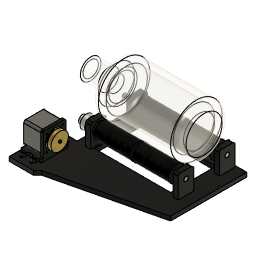
ball-mill v9 (Autodesk Fusion 360 design; units mm, degrees)
Autodesk Fusion 360 part; units mm, degrees
sketch "Sketch1" plane through (0, 0, 0) normal (1, 0, 0) x (0, 1, 0)
  line L0 (17, -21) -> (-17, -21)
  line L1 (-21, -17) -> (-21, 17)
  line L2 (-17, 21) -> (17, 21)
  line L3 (21, 17) -> (21, -17)
  line L4 (21, -21) -> (-21, 21) construction
  line L5 (-21, -21) -> (21, 21) construction
  line L6 (15.5, -15.5) -> (-15.5, -15.5)
  line L7 (-15.5, -15.5) -> (-15.5, 15.5)
  line L8 (-15.5, 15.5) -> (15.5, 15.5)
  line L9 (15.5, 15.5) -> (15.5, -15.5)
  line L10 (15.5, -15.5) -> (-15.5, 15.5) construction
  line L11 (-15.5, -15.5) -> (15.5, 15.5) construction
  circle A0 centre (-15.5, 15.5) radius 1.5
  circle A1 centre (-15.5, -15.5) radius 1.5
  circle A2 centre (15.5, -15.5) radius 1.5
  circle A3 centre (15.5, 15.5) radius 1.5
  arc A4 (-17, 21) -> (-21, 17) centre (-17, 17) ccw
  arc A5 (21, 17) -> (17, 21) centre (17, 17) ccw
  arc A6 (17, -21) -> (21, -17) centre (17, -17) ccw
  arc A7 (-21, -17) -> (-17, -21) centre (-17, -17) ccw
  circle A8 centre (0, 0) radius 11
  circle A9 centre (0, 0) radius 2.5
  dimension "d1" = 42
  dimension "d2" = 42
  dimension "d3" = 31
  dimension "d4" = 3
  dimension "d6" = 360
  dimension "d7" = 4
  dimension "d8" = 22
  dimension "d9" = 5
  constraint horizontal L0
  constraint perpendicular L0 L1
  constraint parallel L0 L2
  constraint parallel L1 L3
  constraint coincident L4 A8.centre
  constraint coincident L5 A8.centre
  constraint coincident A8.centre A9.centre
  constraint horizontal L6
  constraint perpendicular L6 L7
  constraint parallel L6 L8
  constraint parallel L7 L9
  constraint coincident L10 A8.centre
  constraint coincident L11 A8.centre
  constraint coincident L4 L6.start
  constraint coincident L7.end L8.start
  constraint coincident L4.end L2
  constraint coincident L4.end L1
  constraint tangent L2 A4
  constraint tangent L1 A4
  constraint coincident L5.end L2
  constraint coincident L5.end L3
  constraint tangent L2 A5
  constraint tangent L3 A5
  constraint equal A4 A5
  constraint coincident L4.start L3
  constraint coincident L4.start L0
  constraint tangent L3 A6
  constraint tangent L0 A6
  constraint equal A4 A6
  constraint coincident L5.start L0
  constraint coincident L5.start L1
  constraint tangent L0 A7
  constraint tangent L1 A7
  constraint equal A4 A7
  constraint concentric A8 A9
  measures "d1" distance of L4.end L5.end
  measures "d2" distance of L4.start L5.end
  measures "d3" distance of L7.end L8.end
  measures "d4" diameter of A0
  measures "d7" radius of A4
  measures "d8" diameter of A8
  measures "d9" diameter of A9
  measures "d130" radius of L8.end
extrude "Extrude1" add sketch "Sketch1" against normal blind 34 contours L0 L1 L2 L3 A4 A5 A6 A7 | L6 L7 A1 | L6 L7 L8 L9 A0 A1 A2 A3 | L6 L7 A1 | L6 L9 A2 | L6 L9 A2 | L7 L8 A0 | L7 L8 A0 | L8 L9 A3 | L8 L9 A3 | A8 | A9 makes body 1
extrude "Extrude2" cut sketch "Sketch1" against normal blind 5 contours L6 L7 A1 | L6 L7 A1 | L6 L9 A2 | L6 L9 A2 | L7 L8 A0 | L7 L8 A0 | L8 L9 A3 | L8 L9 A3 bodies 1
extrude "Extrude3" add sketch "Sketch1" along normal blind 2 contours A8 | A9 bodies 1
extrude "Extrude4" add sketch "Sketch1" along normal blind 17 contours A9 bodies 1
chamfer "Chamfer1" distance 0.5 angle 45 1 edges at (17, -2.3308, -0.904) on bodies 1
sketch "Sketch2" plane through (0, 0, 0) normal (1, 0, 0) x (0, 1, 0)
  line L0 (22, -22.25) -> (-22, -22.25)
  line L1 (-22, -22.25) -> (-22, 20.25)
  line L2 (-20, 22.25) -> (20, 22.25)
  line L3 (22, 20.25) -> (22, -22.25)
  line L4 (22, -22.25) -> (-22, 22.25) construction
  line L5 (-22, -22.25) -> (22, 22.25) construction
  line L6 (0, 0) -> (-15.5, 15.5) construction
  line L7 (-15.5, -15.5) -> (15.5, 15.5) construction
  circle A0 centre (-15.5, 15.5) radius 1.7
  circle A1 centre (-15.5, -15.5) radius 1.7
  circle A2 centre (15.5, -15.5) radius 1.7
  circle A3 centre (15.5, 15.5) radius 1.7
  circle A4 centre (0, 0) radius 17.5
  line L8 (20, 22.25) -> (22, 20.25)
  line L9 (-22, 20.25) -> (-20, 22.25)
  line L10 (0, -28.25) -> (34, -28.25)
  line L11 (34, -28.25) -> (34, -22.25)
  line L12 (34, -22.25) -> (22, -22.25)
  line L13 (0, -28.25) -> (-34, -28.25)
  line L14 (-34, -22.25) -> (-22, -22.25)
  line L15 (-34, -28.25) -> (-34, -22.25)
  dimension "d19" = 44
  dimension "d20" = 44.5
  dimension "d21" = 31
  dimension "d22" = 3.4
  dimension "d24" = 360
  dimension "d25" = 35
  dimension "d26" = 2
  dimension "d27" = 2
  dimension "d28" = 2
  dimension "d29" = 2
  dimension "d35" = 6
  dimension "d36" = 34
  dimension "d37" = 12
  constraint horizontal L0
  constraint perpendicular L0 L1
  constraint parallel L0 L2
  constraint parallel L1 L3
  constraint coincident L4 L6.start
  constraint coincident L5 L6.start
  constraint coincident L6.start A4.centre
  constraint coincident L6 A4.centre
  constraint coincident L7 L6.start
  constraint coincident L6.end A0.centre
  constraint coincident L5.end L2
  constraint coincident L5.end L3
  constraint coincident L4.end L1
  constraint coincident L4.end L2
  constraint parallel L0 L10
  constraint perpendicular L10 L11
  constraint perpendicular L3 L12
  measures "d19" distance of L4.end L5.end
  measures "d20" distance of L0.end L4.end
  measures "d21" distance of L6.end L7.end
  measures "d22" diameter of A0
  measures "d25" diameter of A4
  measures "d26" distance of L5.end L2.end
  measures "d27" distance of L5.end L3.start
  measures "d28" distance of L4.end L1.end
  measures "d29" distance of L4.end L2.start
  measures "d35" distance of L10.end L11.end
  measures "d36" distance of L10.start L10.end
  measures "d37" distance of L0.start L11.end
ref_plane "WorkPlane1" through (15, 0, 0) normal (1, 0, 0) x (0, 1, 0)
sketch "Sketch3" plane through (15, 0, 0) normal (1, 0, 0) x (0, 1, 0)
  circle A0 centre (0, 0) radius 16.9
  circle A1 centre (0, 0) radius 2.5
  dimension "d31" = 33.8
  dimension "d34" = 5
  constraint coincident A0.centre A1.centre
  measures "d31" diameter of A0
  measures "d34" diameter of A1
extrude "Extrude5" add sketch "Sketch3" against normal blind 7 separate body makes body 2
extrude "Extrude6" add sketch "Sketch2" along normal blind 5 separate body contours L0 L1 L2 L3 L8 L9 makes body 3
extrude "Extrude7" add sketch "Sketch2" along normal blind 5 and the other way blind 34 contours L0 L10 L11 L12 L13 L14 L15 bodies 3
sketch "Sketch4" plane through (0, 0, -22.25) normal (0, 0, 1) x (-1, 0, 0)
  line L0 (0, -22) -> (-5, -22)
  line L1 (-5, -22) -> (-5, -34)
  line L2 (-5, -34) -> (34, -34)
  line L3 (34, -34) -> (34, 34)
  line L4 (34, 34) -> (-5, 34)
  line L5 (-5, 34) -> (-5, 22)
  line L6 (-5, 22) -> (0, 22)
  line L7 (0, 22) -> (0, -22)
  line L8 (-5, -22) -> (34, -22)
  line L9 (34, -22) -> (34, -34)
  line L10 (34, -34) -> (-5, -34)
  line L11 (-5, -34) -> (-5, -26)
  line L12 (5, 0) -> (6, 0)
  line L13 (6, 0) -> (19, 0)
  line L14 (9, -30) -> (9, -29)
  line L15 (12, -26) -> (18, -26)
  line L16 (21, -30) -> (21, -29)
  line L17 (1, -30) -> (1, -29)
  line L18 (-2, -26) -> (-5, -26)
  line L19 (29, -30) -> (29, -29)
  line L20 (32, -26) -> (34, -26)
  circle A0 centre (5, -30) radius 2.25
  circle A1 centre (25, -30) radius 2.25
  arc A2 (1, -30) -> (9, -30) centre (5, -30) ccw
  arc A3 (21, -30) -> (29, -30) centre (25, -30) ccw
  line L21 (25, -34) -> (25, -39)
  line L22 (-5, -34) -> (34, -34)
  line L23 (34, -26) -> (34, -34)
  arc A4 (1, -29) -> (-2, -26) centre (-2, -29) ccw
  arc A5 (12, -26) -> (9, -29) centre (12, -29) ccw
  arc A6 (21, -29) -> (18, -26) centre (18, -29) ccw
  arc A7 (32, -26) -> (29, -29) centre (32, -29) ccw
  line L24 (-5, 34) -> (34, 34)
  line L25 (0, 22) -> (-5, 22)
  line L26 (-5, 22) -> (-5, 34)
  line L27 (-5, 22) -> (34, 22)
  arc A8 (9, 30) -> (1, 30) centre (5, 30) ccw
  line L28 (21, 30) -> (21, 29)
  line L29 (34, 26) -> (34, 34)
  line L30 (1, 30) -> (1, 29)
  arc A9 (18, 26) -> (21, 29) centre (18, 29) ccw
  line L31 (29, 30) -> (29, 29)
  arc A10 (29, 29) -> (32, 26) centre (32, 29) ccw
  line L32 (9, 30) -> (9, 29)
  line L33 (12, 26) -> (18, 26)
  line L34 (34, 22) -> (34, 34)
  arc A11 (9, 29) -> (12, 26) centre (12, 29) ccw
  line L35 (-2, 26) -> (-5, 26)
  line L36 (34, 34) -> (-5, 34)
  line L37 (-5, 34) -> (-5, 26)
  line L38 (-5, 34) -> (34, 34)
  circle A12 centre (5, 30) radius 2.25
  circle A13 centre (25, 30) radius 2.25
  arc A14 (-2, 26) -> (1, 29) centre (-2, 29) ccw
  line L39 (32, 26) -> (34, 26)
  arc A15 (29, 30) -> (21, 30) centre (25, 30) ccw
  point P0 (25, 34)
  dimension "d47" = 4.5
  dimension "d48" = 4.5
  dimension "d49" = 3
  constraint horizontal L8
  constraint vertical L9
  constraint horizontal L10
  constraint vertical L11
  constraint coincident L2.end L3.start
  constraint coincident L0.end L1.start
  constraint perpendicular L7 L12
  constraint perpendicular L7 L13
  constraint tangent L10 A2
  constraint tangent L2 A3
  constraint tangent L14 A2
  constraint tangent L16 A3
  constraint tangent L17 A2
  constraint perpendicular L11 L18
  constraint tangent L19 A3
  constraint coincident L9 L20.end
  constraint concentric A0 A2
  constraint concentric A1 A3
  constraint coincident L2 L21.start
  constraint tangent L18 A4
  constraint tangent L17 A4
  constraint tangent L15 A5
  constraint tangent L14 A5
  constraint equal A4 A5
  constraint tangent L15 A6
  constraint tangent L16 A6
  constraint equal A4 A6
  constraint tangent L19 A7
  constraint tangent L20 A7
  constraint equal A4 A7
  constraint symmetric L0.start L13 L6.end
  constraint symmetric L0.end L13 L5.end
  constraint symmetric L1.end L13 L4.end
  constraint symmetric L2.end L13 L3.end
  constraint symmetric L8.end L13 L27.end
  constraint symmetric L13 L14.start A8.start
  constraint symmetric L13 L16.start L28.start
  constraint symmetric L13 L17.start A8.end
  constraint symmetric L13 L11.end L35.end
  constraint symmetric L13 L19.start L31.start
  constraint symmetric L13 L20.end L29.start
  constraint symmetric L13 A0 A12
  constraint symmetric L13 A1 A13
  constraint symmetric L13 A2 A8
  constraint symmetric L13 A3 A15
  constraint symmetric L13 L21.start P0
  constraint symmetric L13 L18.start L35.start
  constraint symmetric L13 L17.end L30.end
  constraint symmetric L13 A4 A14
  constraint symmetric L13 L15.start L33.start
  constraint symmetric L13 L14.end L32.end
  constraint symmetric L13 A5 A11
  constraint symmetric L13 L15.end A9.start
  constraint symmetric L13 L16.end L28.end
  constraint symmetric L13 A6 A9
  constraint symmetric L13 L19.end L31.end
  constraint symmetric L13 L20.start A10.end
  constraint symmetric L13 A7 A10
  measures "d47" diameter of A0
  measures "d48" diameter of A1
  measures "d49" radius of A4
extrude "Extrude8" cut sketch "Sketch4" against normal blind 10 contours L1 L2 L10 L11 L17 L18 A2 L22 A4 | L2 L3 L9 L10 L19 L20 A3 L22 L23 A7 | L4 L5 L24 L26 A8 L30 L35 L36 L37 L38 A14 | L3 L4 L24 L29 L31 A10 L34 L36 L38 L39 A15 | L2 L10 L14 L15 L16 A2 A3 L22 A5 A6 | L4 L24 A8 L28 A9 L32 L33 A11 L36 L38 A15 bodies 3
extrude "Extrude9" cut sketch "Sketch4" against normal blind 10 contours A0 | A1 | A12 | A13 bodies 3
sketch "Sketch5" plane through (0, 0, -28.25) normal (0, 0, -1) x (1, 0, 0)
  circle A0 centre (-25, -30) radius 2.25
  circle A1 centre (-25, 30) radius 2.25
  circle A2 centre (-5, -30) radius 2.25
  circle A3 centre (-5, 30) radius 2.25
  line L0 (5, 26) -> (2, 26)
  arc A4 (-1, 29) -> (2, 26) centre (2, 29) ccw
  line L1 (-1, 29) -> (-1, 30)
  arc A5 (-1, 30) -> (-9, 30) centre (-5, 30) ccw
  line L2 (-9, 30) -> (-9, 29)
  arc A6 (-12, 26) -> (-9, 29) centre (-12, 29) ccw
  line L3 (-12, 26) -> (-18, 26)
  arc A7 (-21, 29) -> (-18, 26) centre (-18, 29) ccw
  line L4 (-21, 29) -> (-21, 30)
  arc A8 (-21, 30) -> (-29, 30) centre (-25, 30) ccw
  line L5 (-29, 30) -> (-29, 29)
  arc A9 (-32, 26) -> (-29, 29) centre (-32, 29) ccw
  line L6 (-32, 26) -> (-34, 26)
  line L7 (-34, 26) -> (-34, -26)
  line L8 (-34, -26) -> (-32, -26)
  arc A10 (-29, -29) -> (-32, -26) centre (-32, -29) ccw
  line L9 (-29, -29) -> (-29, -30)
  arc A11 (-29, -30) -> (-21, -30) centre (-25, -30) ccw
  line L10 (-21, -30) -> (-21, -29)
  arc A12 (-18, -26) -> (-21, -29) centre (-18, -29) ccw
  line L11 (-18, -26) -> (-12, -26)
  arc A13 (-9, -29) -> (-12, -26) centre (-12, -29) ccw
  line L12 (-9, -29) -> (-9, -30)
  arc A14 (-9, -30) -> (-1, -30) centre (-5, -30) ccw
  line L13 (-1, -30) -> (-1, -29)
  arc A15 (2, -26) -> (-1, -29) centre (2, -29) ccw
  line L14 (2, -26) -> (5, -26)
  line L15 (5, -26) -> (5, 26)
  line L16 (10, 38.1111) -> (-37, 38.1111)
  line L17 (-37, 38.1111) -> (-37, -37.8889)
  line L18 (-37, -37.8889) -> (10, -37.8889)
  line L19 (10, -37.8889) -> (10, 38.1111)
  line L20 (10, 38.1111) -> (-37, -37.8889) construction
  line L21 (-37, 38.1111) -> (10, -37.8889) construction
  line L22 (10, 38.1111) -> (17.9924, 38.1111)
  line L23 (220, -10) -> (220, -157.8889)
  line L24 (220, -157.8889) -> (10, -157.8889)
  line L25 (2.9501, -37.8889) -> (2.9501, -157.8889)
  line L26 (10, -157.8889) -> (2.9501, -157.8889)
  line L27 (-37, -37.8889) -> (-37, -45.8889)
  line L28 (-37, -45.8889) -> (2.9501, -45.8889)
  line L29 (-37, 38.1111) -> (-37, 46.1111)
  line L30 (-37, 46.1111) -> (10, 46.1111)
  line L31 (10, 46.1111) -> (17.9924, 38.1111)
  line L32 (220, -10) -> (17.9924, 38.1111)
  line L33 (180, -137.8889) -> (32.9501, -137.8889)
  line L34 (32.9501, -137.8889) -> (32.9501, -50)
  line L35 (32.9501, -50) -> (180, -50)
  line L36 (180, -50) -> (180, -137.8889)
  point P0 (-13.5, 0.1111)
  point P1 (-5, -30)
  dimension "d54" = 76
  dimension "d55" = 47
  dimension "d61" = 120
  dimension "d110" = 8
  dimension "d112" = 8
  dimension "d123" = 20
  dimension "d124" = 40
  dimension "d125" = 30
  dimension "d126" = 40
  dimension "d134" = 210
  constraint horizontal L16
  constraint perpendicular L16 L17
  constraint parallel L16 L18
  constraint parallel L17 L19
  constraint coincident L20 P0
  constraint coincident L21 P0
  constraint perpendicular L19 L22
  constraint perpendicular L22 L23
  constraint perpendicular L23 L24
  constraint coincident L18 L25.start
  constraint perpendicular L18 L25
  constraint perpendicular L18 L27
  constraint coincident L25 L28.end
  constraint perpendicular L25 L28
  constraint perpendicular L16 L29
  constraint perpendicular L29 L30
  constraint horizontal L33
  constraint vertical L34
  constraint horizontal L35
  constraint vertical L36
  measures "d54" distance of L16.end L17.end
  measures "d55" distance of L17.end L18.end
  measures "d61" distance of L18.end L24.end
  measures "d110" distance of L17.end L27.end
  measures "d112" distance of L16.end L29.end
  measures "d123" distance of L24 L33
  measures "d124" distance of L23.start L35
  measures "d125" distance of L25 L34
  measures "d126" distance of L23 L36
  measures "d134" distance of L23.end L24.end
extrude "Extrude10" add sketch "Sketch5" along normal blind 8 separate body contours L0 A4 L1 A5 L2 A6 L3 A7 L4 A8 L5 A9 L6 L7 L8 A10 L9 A11 L10 A12 L11 A13 L12 A14 L13 A15 L14 L15 | L16 L17 L18 L19 | L18 L19 L22 L23 L24 L25 L26 L32 | L16 L22 L29 L30 L31 | L18 L25 L27 L28 makes body 4
sketch "Sketch6" plane through (0, 0, -28.25) normal (0, 0, 1) x (-1, 0, 0)
  circle A0 centre (25, 30) radius 2.25
  circle A1 centre (5, 30) radius 2.25
  circle A2 centre (5, -30) radius 2.25
  circle A3 centre (25, -30) radius 2.25
  line L0 (-220, -10) -> (-220, -157.8889)
  line L1 (-220, -157.8889) -> (-2.9501, -157.8889)
  line L2 (-2.9501, -157.8889) -> (-2.9501, -45.8889)
  line L3 (37, -45.8889) -> (37, 46.1111)
  line L4 (-35, 0) -> (10, 0)
  line L5 (-230, -60) -> (70, -60)
  line L6 (-235, -110) -> (40, -110)
  line L7 (-15, 0) -> (-15, -175)
  line L8 (-8, -37.8889) -> (-8, -175)
  line L9 (-15, -60) -> (-35, -60)
  line L10 (-30, -60) -> (-30, -45)
  line L11 (-30, -45) -> (-20, -45)
  line L12 (-20, -45) -> (-20, -60)
  line L13 (-30, -60) -> (-30, -75)
  line L14 (-30, -75) -> (-20, -75)
  line L15 (-20, -75) -> (-20, -60)
  line L16 (-235.1894, -85) -> (34.547, -85)
  line L17 (-30, -110) -> (-30, -125)
  line L18 (-30, -125) -> (-20, -125)
  line L19 (-20, -125) -> (-20, -110)
  line L20 (-20, -95) -> (-20, -110)
  line L21 (-30, -110) -> (-30, -95)
  line L22 (-30, -95) -> (-20, -95)
  line L23 (37, 46.1111) -> (-10, 46.1111)
  line L24 (-10, 46.1111) -> (-17.9924, 38.1111)
  line L25 (-2.9501, -45.8889) -> (37, -45.8889)
  line L26 (-17.9924, 38.1111) -> (-220, -10)
  line L27 (-180, -50) -> (-32.9501, -50)
  line L28 (-32.9501, -50) -> (-32.9501, -137.8889)
  line L29 (-32.9501, -137.8889) -> (-180, -137.8889)
  line L30 (-180, -137.8889) -> (-180, -50)
  dimension "d64" = 60
  dimension "d65" = 50
  dimension "d66" = 7
  dimension "d67" = 15
  dimension "d68" = 10
  dimension "d70" = 50
  constraint horizontal L4
  constraint perpendicular L0 L5
  constraint horizontal L6
  constraint coincident L4 L7.start
  constraint perpendicular L4 L7
  constraint perpendicular L1 L8
  constraint coincident L5 L9.start
  constraint coincident L7 L9.start
  constraint coincident L5 L9.end
  constraint perpendicular L7 L9
  constraint coincident L5 L10.start
  constraint perpendicular L9 L10
  constraint perpendicular L10 L11
  constraint coincident L9 L12.end
  constraint perpendicular L11 L12
  constraint symmetric L5 L10.start L13.start
  constraint symmetric L5 L10.end L13.end
  constraint symmetric L5 L11.end L14.end
  constraint symmetric L5 L12.end L15.end
  constraint perpendicular L8 L16
  constraint symmetric L10.start L16 L17.start
  constraint symmetric L10.end L16 L17.end
  constraint symmetric L11.end L16 L18.end
  constraint symmetric L12.end L16 L19.end
  constraint symmetric L13.end L16 L21.end
  constraint symmetric L14.end L16 L20.start
  measures "d64" distance of L4 L5
  measures "d65" distance of L5 L6
  measures "d66" distance of L7 L8
  measures "d67" distance of L10.start L10.end
  measures "d68" distance of L10.end L11.end
extrude "Extrude11" add sketch "Sketch6" along normal blind 43 separate body contours L5 L9 L10 L11 L12 | L5 L9 L13 L14 L15 | L6 L20 L21 L22 | L6 L17 L18 L19 makes body 5 at (30, 65, -13.9167) makes body 6 at (30, 115, -13.9167)
sketch "Sketch7" plane through (30, 0, 0) normal (1, 0, 0) x (0, 1, 0)
  line L0 (75, -28.25) -> (75, 14.75)
  line L1 (75, 14.75) -> (45, 14.75)
  line L2 (45, 14.75) -> (45, -28.25)
  line L3 (36, -0.25) -> (89, -0.25)
  line L4 (60, 25) -> (60, -13)
  circle A0 centre (60, -0.25) radius 11.5
  circle A1 centre (60, -0.25) radius 11
  line L5 (89, -0.25) -> (136, -0.25)
  line L6 (110, 21) -> (110, -16)
  line L7 (95, -28.25) -> (95, 14.75)
  circle A2 centre (110, -0.25) radius 11.5
  circle A3 centre (110, -0.25) radius 11
  circle A4 centre (60, -0.25) radius 4.5
  circle A5 centre (60, -0.25) radius 4
  circle A6 centre (110, -0.25) radius 4.5
  circle A7 centre (110, -0.25) radius 4
  line L8 (45, -28.25) -> (75, -28.25)
  dimension "d73" = 15
  dimension "d74" = 15
  dimension "d75" = 23
  dimension "d76" = 22
  dimension "d79" = 15
  dimension "d80" = 23
  dimension "d81" = 22
  dimension "d84" = 9
  dimension "d85" = 8
  dimension "d86" = 9
  dimension "d87" = 8
  constraint horizontal L3
  constraint perpendicular L3 L4
  constraint coincident L3 A0.centre
  constraint coincident L4 A0.centre
  constraint concentric A0 A1
  constraint parallel L3 L5
  constraint perpendicular L5 L6
  constraint coincident L6 A2.centre
  constraint coincident L5 A2.centre
  constraint concentric A2 A3
  constraint concentric A1 A4
  constraint concentric A1 A5
  constraint concentric A2 A6
  constraint concentric A3 A7
  measures "d73" distance of L1 L3
  measures "d74" distance of L2 L4
  measures "d75" diameter of A0
  measures "d76" diameter of A1
  measures "d79" distance of L6 L7
  measures "d80" diameter of A2
  measures "d81" diameter of A3
  measures "d84" diameter of A4
  measures "d85" diameter of A5
  measures "d86" diameter of A6
  measures "d87" diameter of A7
extrude "Extrude12" cut sketch "Sketch7" against normal blind 7 contours L3 L4 A0 A1 | L3 L4 A0 A1 | L3 L4 A1 A4 | L3 L4 A1 A4 | L3 L4 A0 A1 | L3 L4 A0 A1 | L3 L4 A4 A5 | L3 L4 A4 A5 | L3 L4 A1 A4 | L3 L4 A1 A4 | L3 L4 A5 | L3 L4 A5 | L3 L4 A4 A5 | L3 L4 A4 A5 | L3 L4 A5 | L3 L4 A5 | L5 L6 A6 A7 | L5 L6 A7 | L5 L6 A7 | L5 L6 A6 A7 | L5 L6 A3 A6 | L5 L6 A3 A6 | L5 L6 A7 | L5 L6 A7 | L5 L6 A6 A7 | L5 L6 A6 A7 | L5 L6 A2 A3 | L5 L6 A2 A3 | L5 L6 A3 A6 | L5 L6 A3 A6 | L5 L6 A2 A3 | L5 L6 A2 A3 bodies 6 5 4
extrude "Extrude13" cut sketch "Sketch7" against normal blind 12 contours L3 L4 A4 A5 | L3 L4 A4 A5 | L3 L4 A5 | L3 L4 A5 | L3 L4 A4 A5 | L3 L4 A4 A5 | L3 L4 A5 | L3 L4 A5 | L5 L6 A6 A7 | L5 L6 A7 | L5 L6 A7 | L5 L6 A6 A7 | L5 L6 A7 | L5 L6 A7 | L5 L6 A6 A7 | L5 L6 A6 A7 bodies 6 4 5
extrude "Extrude14" add sketch "Sketch7" against normal blind 7 separate body contours L3 L4 A1 A4 | L3 L4 A1 A4 | L3 L4 A4 A5 | L3 L4 A4 A5 | L3 L4 A1 A4 | L3 L4 A1 A4 | L3 L4 A4 A5 | L3 L4 A4 A5 | L5 L6 A6 A7 | L5 L6 A6 A7 | L5 L6 A3 A6 | L5 L6 A3 A6 | L5 L6 A6 A7 | L5 L6 A6 A7 | L5 L6 A3 A6 | L5 L6 A3 A6 makes body 7 at (25.3333, 70.9453, -1.3452) makes body 8 at (25.3333, 120.9453, -1.3452)
fillet "Fillet1" radius 4 4 edges at (25, 45, 14.75) (25, 75, 14.75) (25, 95, 14.75) (25, 125, 14.75) on bodies 5 6
extrude "Extrude15" add sketch "Sketch7" along normal blind 170 and the other way blind 30 separate body contours L3 L4 A5 | L3 L4 A5 | L3 L4 A5 | L3 L4 A5 | L5 L6 A7 | L5 L6 A7 | L5 L6 A7 | L5 L6 A7 makes body 9 at (143.3333, 63.9955, -0.4403) makes body 10 at (143.3333, 113.9955, -0.4403)
sketch "Sketch8" plane through (20, 0, 0) normal (-1, 0, 0) x (0, -1, 0)
  circle A0 centre (-60, -0.25) radius 4.5
  arc A1 (-71, 14.75) -> (-75, 10.75) centre (-71, 10.75) ccw
  line L0 (-75, 10.75) -> (-75, -28.25)
  line L1 (-45, -28.25) -> (-45, 10.75)
  arc A2 (-45, 10.75) -> (-49, 14.75) centre (-49, 10.75) ccw
  line L2 (-49, 14.75) -> (-71, 14.75)
  circle A3 centre (-60, -0.25) radius 12.75
  circle A4 centre (-60, -0.25) radius 7.5
  circle A5 centre (-60, -0.25) radius 4
  line L3 (-75, -28.25) -> (-45, -28.25)
  dimension "d98" = 25.5
  dimension "d99" = 15
  dimension "d102" = 8
  constraint concentric A0 A3
  constraint concentric A3 A4
  constraint concentric A3 A5
  measures "d98" diameter of A3
  measures "d99" diameter of A4
  measures "d102" diameter of A5
extrude "Extrude16" add sketch "Sketch8" along normal blind 9 separate body contours A3 makes body 11
extrude "Extrude17" add sketch "Sketch8" along normal blind 17 separate body contours A0 | A4 makes body 12
combine "Combine1" operation add target body 12 tool bodies 11
move_body "Move1" bodies 12 to x (1, 0, 0) y (0, 1, 0) z (0, 0, 1) at (-4, 0, 0)
copy_body "CopyPasteBodies2" bodies 5 makes body 13
move_body "Move3" bodies 13 to x (-1, 0, 0) y (0, -1, 0) z (0, 0, 1) at (60, 120, 0)
move_body "Move4" bodies 13 to x (1, 0, 0) y (0, 1, 0) z (0, 0, 1) at (160, 0, 0)
copy_body "CopyPasteBodies3" bodies 6 makes body 14
move_body "Move5" bodies 14 to x (-1, 0, 0) y (0, -1, 0) z (0, 0, 1) at (60, 220, 0)
move_body "Move6" bodies 14 to x (1, 0, 0) y (0, 1, 0) z (0, 0, 1) at (160, 0, 0)
copy_body "CopyPasteBodies4" bodies 7 makes body 15
move_body "Move7" bodies 15 to x (1, 0, 0) y (0, 1, 0) z (0, 0, 1) at (167, 0, 0)
copy_body "CopyPasteBodies5" bodies 8 makes body 16
move_body "Move8" bodies 16 to x (1, 0, 0) y (0, 1, 0) z (0, 0, 1) at (167, 0, 0)
sketch "Sketch10" plane through (0, 0, -36.25) normal (0, 0, -1) x (1, 0, 0)
  circle A0 centre (-25, 30) radius 2.25
  circle A1 centre (-5, 30) radius 2.25
  circle A2 centre (-5, -30) radius 2.25
  circle A3 centre (-25, -30) radius 2.25
  line L0 (-37, 46.1111) -> (-37, -45.8889)
  line L1 (2.9501, -45.8889) -> (2.9501, -157.8889)
  line L2 (2.9501, -157.8889) -> (220, -157.8889)
  line L3 (220, -157.8889) -> (220, -10)
  line L4 (-2.75, -25) -> (-2.75, -35)
  line L5 (-7.25, -35) -> (-7.25, -25)
  line L6 (-37, -45.8889) -> (2.9501, -45.8889)
  line L7 (17.9924, 38.1111) -> (10, 46.1111)
  line L8 (10, 46.1111) -> (-37, 46.1111)
  line L9 (-0.25, -25) -> (-0.25, -35)
  line L10 (-9.75, -35) -> (-9.75, -25)
  arc A4 (-0.25, -25) -> (-9.75, -25) centre (-5, -25) ccw
  arc A5 (-9.75, -35) -> (-0.25, -35) centre (-5, -35) ccw
  arc A6 (-7.25, -35) -> (-2.75, -35) centre (-5, -35) ccw
  arc A7 (-2.75, -25) -> (-7.25, -25) centre (-5, -25) ccw
  arc A8 (-29.75, -35) -> (-20.25, -35) centre (-25, -35) ccw
  line L11 (-27.25, -35) -> (-27.25, -25)
  arc A9 (-27.25, -35) -> (-22.75, -35) centre (-25, -35) ccw
  line L12 (-22.75, -25) -> (-22.75, -35)
  line L13 (-20.25, -25) -> (-20.25, -35)
  line L14 (-29.75, -35) -> (-29.75, -25)
  arc A10 (-20.25, -25) -> (-29.75, -25) centre (-25, -25) ccw
  arc A11 (-22.75, -25) -> (-27.25, -25) centre (-25, -25) ccw
  arc A12 (-9.75, 25) -> (-0.25, 25) centre (-5, 25) ccw
  line L15 (-7.25, 25) -> (-7.25, 35)
  arc A13 (-7.25, 25) -> (-2.75, 25) centre (-5, 25) ccw
  line L16 (-2.75, 35) -> (-2.75, 25)
  line L17 (-0.25, 35) -> (-0.25, 25)
  line L18 (-9.75, 25) -> (-9.75, 35)
  arc A14 (-0.25, 35) -> (-9.75, 35) centre (-5, 35) ccw
  arc A15 (-2.75, 35) -> (-7.25, 35) centre (-5, 35) ccw
  arc A16 (-29.75, 25) -> (-20.25, 25) centre (-25, 25) ccw
  line L19 (-27.25, 25) -> (-27.25, 35)
  arc A17 (-27.25, 25) -> (-22.75, 25) centre (-25, 25) ccw
  line L20 (-22.75, 35) -> (-22.75, 25)
  line L21 (-20.25, 35) -> (-20.25, 25)
  line L22 (-29.75, 25) -> (-29.75, 35)
  arc A18 (-20.25, 35) -> (-29.75, 35) centre (-25, 35) ccw
  arc A19 (-22.75, 35) -> (-27.25, 35) centre (-25, 35) ccw
  line L23 (220, -10) -> (17.9924, 38.1111)
  line L24 (32.9501, -50) -> (180, -50)
  line L25 (180, -50) -> (180, -137.8889)
  line L26 (180, -137.8889) -> (32.9501, -137.8889)
  line L27 (32.9501, -137.8889) -> (32.9501, -50)
  point P0 (-5, -30)
  point P1 (-5, -30)
  dimension "d108" = 4.5
  dimension "d109" = 10
  dimension "d113" = 9.5
  dimension "d114" = 10
  dimension "d117" = -20
  dimension "d118" = 60
  constraint parallel L4 L5
  constraint coincident P1 P0
  constraint parallel L9 L10
  constraint concentric A4 A7
  measures "d108" distance of L4.end L5.start
  measures "d109" distance of L4.start L4.end
  measures "d113" distance of L9.end L10.start
  measures "d114" distance of L9.start L9.end
extrude "Extrude18" cut sketch "Sketch10" against normal blind 8 contours A0 L19 A17 L20 | A0 L19 L20 A19 | A1 L15 A13 L16 | A1 L15 L16 A15 | A2 L4 L5 A6 | A2 L4 L5 A7 | A3 L11 A9 L12 | A3 L11 L12 A11 bodies 4
extrude "Extrude19" cut sketch "Sketch10" against normal blind 4.5 contours L9 L10 A4 A5 | A8 L13 L14 A10 | A12 L17 L18 A14 | A16 L21 L22 A18 bodies 4
sketch "Sketch11" plane through (0, 0, 0) normal (0, 0, 1) x (1, 0, 0)
  line L0 (0, 0) -> (-10, 0)
  line L1 (-155, -50) -> (-15, -50)
  line L2 (0, -35) -> (0, 0)
  line L3 (-220, -15) -> (-220, -20)
  line L4 (-220, -20) -> (-185, -20)
  line L5 (-10, 0) -> (-10, -30)
  line L6 (-20, -40) -> (-150, -40)
  line L7 (-160, -30) -> (-160, -25)
  arc A0 (-170, -35) -> (-155, -50) centre (-155, -35) ccw
  arc A1 (-15, -50) -> (0, -35) centre (-15, -35) ccw
  arc A2 (-170, -35) -> (-185, -20) centre (-185, -35) ccw
  line L8 (-220, -15) -> (-170, -15)
  arc A3 (-160, -25) -> (-170, -15) centre (-170, -25) ccw
  arc A4 (-160, -30) -> (-150, -40) centre (-150, -30) ccw
  arc A5 (-20, -40) -> (-10, -30) centre (-20, -30) ccw
  point P0 (-170, -50)
  point P1 (0, -50)
  dimension "d127" = 170
  dimension "d129" = 50
  dimension "d130" = 15
  dimension "d131" = 10
  dimension "d133" = 140
  constraint horizontal L0
  constraint horizontal L1
  constraint vertical L2
  constraint coincident L0.start L2.end
  constraint vertical L3
  constraint horizontal L4
  constraint perpendicular L0 L5
  constraint perpendicular L5 L6
  constraint perpendicular L0 L7
  constraint coincident P0 L1
  constraint tangent L1 A0
  constraint coincident P1 L1
  constraint coincident P1 L2
  constraint tangent L1 A1
  constraint tangent L2 A1
  constraint equal A0 A1
  constraint tangent L4 A2
  constraint equal A0 A2
  constraint coincident A0.start A2.start
  constraint perpendicular L7 L8
  constraint tangent L7 A3
  constraint tangent L8 A3
  constraint tangent L6 A4
  constraint tangent L7 A4
  constraint equal A3 A4
  constraint tangent L6 A5
  constraint tangent L5 A5
  constraint equal A3 A5
  measures "d127" distance of P0 P1
  measures "d129" distance of L0.start P1
  measures "d130" radius of A0
  measures "d131" radius of A3
  measures "d133" distance of L1.start L1.end
revolve "Revolve1" add sketch "Sketch11" angle 360 about axis through (1.75, 0, 0) along (1, 0, 0) separate body makes body 17
move_body "Move9" bodies 17 to x (1, 0, 0) y (0, 1, 0) z (0, 0, 1) at (195, 0, 60)
move_body "Move12" bodies 16 14 10 8 6 to x (1, 0, 0) y (0, 1, 0) z (0, 0, 1) at (0, 30, 0)
sketch "Sketch12" plane through (7, 0, 0) normal (-1, 0, 0) x (0, -1, 0)
  circle A0 centre (-60, -0.25) radius 7.5
  circle A1 centre (-60, -0.25) radius 12.75
  circle A2 centre (-60, -0.25) radius 16
  circle A3 centre (-60, -0.25) radius 3.85
  dimension "d135" = 32
  dimension "d136" = 7.7
  constraint concentric A0 A2
  constraint concentric A2 A3
  measures "d135" diameter of A2
  measures "d136" diameter of A3
extrude "Extrude20" add sketch "Sketch12" along normal blind 70 separate body contours A0 | A1 | A2 makes body 18
move_body "Move14" bodies 18 to x (1, 0, 0) y (0, 1, 0) z (0, 0, 1) at (100, 0, 0)
copy_body "CopyPasteBodies6" bodies 18 makes body 19
move_body "Move15" bodies 19 to x (1, 0, 0) y (0, 1, 0) z (0, 0, 1) at (75, 0, 0)
copy_body "CopyPasteBodies7" bodies 19 18 makes body 20 makes body 21
move_body "Move16" bodies 20 21 to x (1, 0, 0) y (0, 1, 0) z (0, 0, 1) at (0, 80, 0)
move_body "Move18" bodies 17 to x (1, 0, 0) y (0, 1, 0) z (0, 0, 1) at (0, 100, -8)
combine "Combine2" operation add target body 4 tool bodies 5 6 13 14
equation "d27 = d26"
equation "d29 = d28"
named bodies: "stepped-motor", "motor-braket", "base", "bearing01", "bearing02", "bar01", "bar02", "bearing-holder01", "bearing-holder02", "bearing-holder01 (1)", "bearing-holder02 (1)", "bearing01 (1)", "bearing02 (1)", "bottle", "rubber01", "rabber01", "rubber02", "rabber02", "rabber01 (1)", "rubber04", "rubber03"
